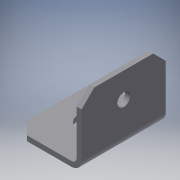
# Autodesk Inventor part: Part107
Saved by Autodesk Inventor 2016 (Build 200138000, 138)
## iProperties
Created: 2018-11-14
Part Number: Part107
Material: Generic
Document SubType Name: Sheet Metal
Designer: hovm
Density: 1 g/cm^3
Sheet Metal Rule: Default_mm
Appearance: Default
Author: hovm
Autodesk Inventor part; units mm, degrees
ref_plane "YZ Plane" through (0, 0, 0) normal (1, 0, 0) x (0, 1, 0)
ref_plane "XZ Plane" through (0, 0, 0) normal (0, 1, 0) x (-1, 0, 0)
ref_plane "XY Plane" through (0, 0, 0) normal (0, 0, 1) x (1, 0, 0)
sketch "Sketch1" plane through (0, 0, 0) normal (0, 0, 1) x (1, 0, 0)
  line L0 (-8, -10) -> (8, -10)
  line L1 (8, -10) -> (8, 10)
  line L2 (8, 10) -> (-8, 10)
  line L3 (-8, 10) -> (-8, -10)
  line L4 (-8, -10) -> (8, 10) construction
  line L5 (8, -10) -> (-8, 10) construction
  point P0 (0, 0)
  dimension "d0" = 16
  dimension "d1" = 20
  measures "d0" distance of L1.end L2.end
  measures "d1" distance of L0.end L1.end
extrude "Plate1" add sketch "Sketch1" along normal blind 1.2
sketch "Sketch2" plane through (6.8, 10, 0) normal (1, 0, 0) x (0, 1, 0)
  line L0 (-20, 0) -> (0, 0)
  line L1 (0, 0) -> (0, 16)
  line L2 (0, 16) -> (-20, 16)
  line L3 (-20, 16) -> (-20, 0)
  constraints: 6 end point, 1 horizontal, 1 perpendicular, 1 vertical
edge flange "Flange1" height 16 angle 90 thickness 1.2 bend radius 1.2 thickness toward (1, 0, 0) relief tear relief width 1.2 relief depth 0.6 edges at (8, 0, 1.2) wall of the first edge with corners at (6.8, -10, 0) (6.8, 10, 0) (6.8, 10, 16) (6.8, -10, 16)
bend "Bend1"
corner "Corner1"
chamfer "Corner Chamfer1" distance 3 angle 45 4 edges at (-8, 10, 0.6) (-8, -10, 0.6) (7.4, -10, 16) (7.4, 10, 16)
sketch "Sketch3" plane through (6.8, -10, 2.4) normal (-1, 0, 0) x (0, 0, 1)
  line L0 (13.6, 3) -> (13.6, 17) projected
  line L1 (-2.4, 17) -> (-2.4, 3) projected
  point P0 (-2.4, 10)
  point P1 (7.6, 10)
  point P2 (-2.4, 10)
  dimension "d16" = 6
  constraints: 1 horizontal alignment, 1 midpoint
  measures "d16" distance from line of L0 point (7.6, 10)
hole "Hole1" at (6.8, 0, 10) direction (1, 0, 0) diameter 3 depth 1.2 tip angle 118
sketch "Sketch4" plane through (0, 0, 1.2) normal (0, 0, 1) x (1, 0, 0)
  circle A0 centre (-0.5392, 0) radius 2.1 construction
  circle A1 centre (-0.5392, 0) radius 2.5
  point P0 (0, 0)
  dimension "d24" = 0.4
  constraints: 1 centre point
  measures "d24" radial gap between concentric circles of A0 A1
extrude "Cut1" cut sketch "Sketch4" against normal blind 1.2
equation "\"d22\" = Thickness"
equation "\"d25\" = Thickness"
equation "\"d3\" = BendReliefWidth"
equation "\"d4\" = BendReliefDepth"
equation "\"d5\" = MinimumRemnant"
equation "\"d6\" = BendRadius"
equation "\"d9\" = BendRadius"
equation "\"d10\" = CornerReliefSize"
equation "\"d11\" = GapSize"
equation "\"d12\" = JacobiRadiusSize"
equation "\"BendRadius\" = Thickness"
equation "\"BendReliefWidth\" = Thickness"
equation "\"BendReliefDepth\" = 0.5 * Thickness"
equation "\"CornerReliefSize\" = 4 * Thickness"
equation "\"MinimumRemnant\" = 2 * Thickness"
equation "\"TransitionRadius\" = BendRadius"
equation "\"JacobiRadiusSize\" = BendRadius"
equation "\"GapSize\" = Thickness"
equation "\"d2\" = BendRadius"
equation "\"Thickness\" = 1.2"
body "Solid1"
